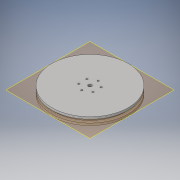
# Autodesk Inventor part: WoodPully
Saved by Autodesk Inventor 2016 SP1 (Build 200210100, 210)
## iProperties
Created: 2016-01-27
Part Number: WoodPully
Material: Generic
Document SubType Name: Modeling
Designer: steele
Density: 1 g/cm^3
Appearance: Default
Author: steele
Autodesk Inventor part; units mm, degrees
ref_plane "YZ Plane" through (0, 0, 0) normal (1, 0, 0) x (0, 1, 0)
ref_plane "XY Plane" through (0, 0, 0) normal (0, 0, 1) x (1, 0, 0)
sketch "Sketch1" plane through (0, 0, 0) normal (0, 1, 0) x (-1, 0, 0)
  circle A0 centre (0, 0) radius 101.6
  dimension "d0" = 203.2
  constraints: 1 centre point, 1 coincident
  measures "d0" diameter of A0
extrude "Extrusion1" add sketch "Sketch1" along normal mid plane 9.525
sketch "Sketch2" plane through (0, 4.7625, 0) normal (0, 1, 0) x (1, 0, 0)
  circle A0 centre (0, 0) radius 111.125
  dimension "d3" = 222.25
  constraints: 1 centre point, 1 coincident
  measures "d3" diameter of A0
extrude "Extrusion2" add sketch "Sketch2" along normal blind 6.35
mirror "Mirror1" about plane through (0, 0, 0) normal (0, 1, 0) of "Extrusion2"
sketch "Sketch4" plane through (0, 11.1125, 0) normal (0, 1, 0) x (1, 0, 0)
  circle A0 centre (0, 23.8125) radius 2.54
  circle A1 centre (-20.6222, 11.9063) radius 2.54
  circle A2 centre (-20.6222, -11.9062) radius 2.54
  circle A3 centre (0, -23.8125) radius 2.54
  circle A4 centre (20.6222, -11.9063) radius 2.54
  circle A5 centre (20.6222, 11.9062) radius 2.54
  point P0 (0, 0)
  dimension "d6" = 5.08
  dimension "d7" = 23.8125
  dimension "d10" = 360
  constraints: 6 centre point, 13 other
  measures "d6" diameter of A0
  measures "d7" distance of A0.centre point (0, 0)
extrude "Extrusion3" cut sketch "Sketch4" against normal through all
sketch "Sketch5" plane through (0, 11.1125, 0) normal (0, 1, 0) x (1, 0, 0)
  circle A0 centre (0, 0) radius 5
  dimension "d14" = 10
  constraints: 1 centre point, 1 coincident
  measures "d14" diameter of A0
extrude "Extrusion4" cut sketch "Sketch5" against normal through all
equation "\"d0\" = innerDiam"
equation "\"d1\" = innerWidth"
equation "\"d3\" = outerDiam"
equation "\"d4\" = outerWidth"
equation "\"d12\" = outerWidth"
equation "\"d15\" = outerWidth"
equation "\"innerDiam\" = 203.2"
equation "\"innerRadius\" = 0.5 * innerDiam"
equation "\"outerDiam\" = 2 * outerRadius"
equation "\"innerWidth\" = 9.525"
equation "\"outerWidth\" = 6.35"
equation "\"outerRadius\" = 111.125"
body "Solid1"
